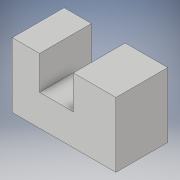
# Autodesk Inventor part: test print
Saved by Autodesk Inventor 2017 (Build 210142000, 142)
## iProperties
Created: 2018-02-12
Part Number: test print
Material: Generic
Document SubType Name: Modeling
Designer: Tripl_000
Density: 1 g/cm^3
Appearance: Default
Author: Tripl_000
Autodesk Inventor part; units mm, degrees
ref_plane "YZ Plane" through (0, 0, 0) normal (1, 0, 0) x (0, 1, 0)
ref_plane "XZ Plane" through (0, 0, 0) normal (0, 1, 0) x (-1, 0, 0)
ref_plane "XY Plane" through (0, 0, 0) normal (0, 0, 1) x (1, 0, 0)
sketch "Sketch1" plane through (0, 0, 0) normal (0, 1, 0) x (-1, 0, 0)
  line L0 (20, 10) -> (-20, 10)
  line L1 (-20, 10) -> (-20, -10)
  line L2 (-20, -10) -> (20, -10)
  line L3 (20, -10) -> (20, 10)
  line L4 (20, 10) -> (-20, -10) construction
  line L5 (-20, 10) -> (20, -10) construction
  point P0 (0, 0)
  dimension "d0" = 20
  dimension "d1" = 40
  constraints: 12 end point, 2 midpoint, 2 parallel, 1 horizontal, 1 perpendicular
  measures "d0" distance of L2.end L0.start
  measures "d1" distance of L1.end L2.end
extrude "Extrusion1" add sketch "Sketch1" along normal blind 25
sketch "Sketch2" plane through (-20, 0, 10) normal (0, 0, 1) x (1, 0, 0)
  line L0 (0, 25) -> (40, 25) projected
  line L1 (10.5659, 25) -> (23.5659, 25)
  line L2 (23.5659, 25) -> (23.5659, 12)
  line L3 (23.5659, 12) -> (10.5659, 12)
  line L4 (10.5659, 12) -> (10.5659, 25)
  point P0 (20, 0)
  dimension "d4" = 13
  dimension "d5" = 13
  constraints: 8 end point, 2 parallel, 1 horizontal, 1 perpendicular, 1 point on line
  measures "d4" distance between parallel lines of L2 L4
  measures "d5" distance between parallel lines of L0 L3
extrude "Extrusion2" cut sketch "Sketch2" against normal through all
body "Solid1"
